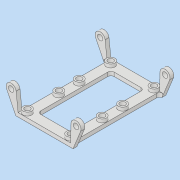
# Autodesk Inventor part: RelayHolderREV2
Saved by Autodesk Inventor 2017.3 (Build 213256000, 256)
## iProperties
Created: 2019-02-24
Part Number: RelayHolderREV2
Material: ABS Plastic
Document SubType Name: Modeling
Designer: Derek Wider
Density: 1.06 g/cm^3
Appearance: Smooth - White
Author: Derek Wider
Autodesk Inventor part; units mm, degrees
ref_plane "YZ Plane" through (0, 0, 0) normal (1, 0, 0) x (0, 1, 0)
ref_plane "XZ Plane" through (0, 0, 0) normal (0, 1, 0) x (-1, 0, 0)
ref_plane "XY Plane" through (0, 0, 0) normal (0, 0, 1) x (1, 0, 0)
sketch "Sketch1" plane through (0, 0, 0) normal (0, 1, 0) x (-1, 0, 0)
  line L0 (0, 0) -> (34, 0)
  line L1 (34, 0) -> (34, -60)
  line L2 (34, -60) -> (0, -60)
  line L3 (0, -60) -> (0, 0)
  dimension "d0" = 34
  dimension "d1" = 60
  constraints: 8 end point, 2 parallel, 1 horizontal, 1 perpendicular
  measures "d0" distance of L1.end L2.end
  measures "d1" distance of L0.end L1.end
extrude "Extrusion1" add sketch "Sketch1" along normal blind 2.5
sketch "Sketch4" plane through (-34, 0, 0) normal (0, 0, 1) x (1, 0, 0)
  circle A0 centre (-4.5, 13.5) radius 1.75
  circle A1 centre (-4.5, 13.5) radius 3.25
  circle A2 centre (37.41, 13.5) radius 1.75
  circle A3 centre (37.41, 13.5) radius 3.25
  line L0 (0, 0) -> (0, 2.5) projected
  line L1 (0, 2.5) -> (34, 2.5) projected
  line L2 (0, 2.5) -> (-1.2701, 13.8611)
  line L3 (34, 0) -> (0, 0) projected
  line L4 (0, 0) -> (-1.5, 0)
  line L5 (-1.5, 0) -> (-7.4181, 12.0691)
  line L6 (34, 2.5) -> (34.1603, 13.5472)
  line L7 (34, 0) -> (35.5, 0)
  line L8 (35.5, 0) -> (40.4267, 12.2908)
  line L9 (34, 0) -> (34, 2.5) projected
  line L10 (34, 2.5) -> (34, 0)
  dimension "d4" = 3.5
  dimension "d5" = 6.5
  dimension "d6" = 4.5
  dimension "d7" = 41.91
  dimension "d8" = 11
  dimension "d9" = 1.5
  dimension "d10" = 1.5
  constraints: 14 end point, 4 centre point, 4 point on circle, 4 tangent, 2 coincident, 2 equal radius, 1 collinear, 1 horizontal, 1 horizontal alignment, 1 point on line
  measures "d4" diameter of A0
  measures "d5" diameter of A1
  measures "d6" distance from line of L0 A0.centre
  measures "d7" distance of A0.centre A2.centre
  measures "d8" distance from line of A0.centre L1
  measures "d9" distance of L0.start L4.end
  measures "d10" distance of L3.start L7.end
extrude "Extrusion2" add sketch "Sketch4" against normal blind 2.5 contours A1 | A1 L2 L0 L4 L5 | L6 A3 L8 L7 L9 | A3
pattern_linear "Rectangular Pattern1" count 2 spacing 57.5 along (0, 0, -1) of "Extrusion2"
hole "Hole1" at (-31, 2.5, -3) direction (0, -1, 0) diameter 3.5 end through all
sketch "Sketch7" plane through (0, 2.5, 0) normal (0, 1, 0) x (1, 0, 0)
  circle A0 centre (-31, 3) radius 1.75 projected
  circle A1 centre (-31, 3) radius 2.75
  point P0 (0, 0)
  dimension "d37" = 5.5
  constraints: 1 centre point, 1 coincident
  measures "d37" diameter of A1
extrude "Extrusion3" add sketch "Sketch7" along normal blind 2.2
pattern_linear "Rectangular Pattern2" count 2 spacing 28 along (1, 0, 0) count 2 spacing 20.3 along (0, 0, -1) of "Hole1", "Extrusion3"
pattern_linear "Rectangular Pattern3" count 2 spacing 33.5 along (0, 0, -1) of "Rectangular Pattern2", "Extrusion3", "Hole1"
sketch "Sketch8" plane through (0, 2.5, 0) normal (0, 1, 0) x (1, 0, 0)
  circle A0 centre (-3, 56.8) radius 2.75 projected
  circle A1 centre (-31, 56.8) radius 2.75 projected
  circle A2 centre (-3, 36.5) radius 2.75 projected
  circle A3 centre (-31, 36.5) radius 2.75 projected
  circle A4 centre (-3, 23.3) radius 2.75 projected
  circle A5 centre (-31, 23.3) radius 2.75 projected
  circle A6 centre (-3, 3) radius 2.75 projected
  circle A7 centre (-31, 3) radius 2.75 projected
  line L0 (-34, 0) -> (0, 0) projected
  line L1 (0, 0) -> (0, 2.5) projected
  line L2 (0, 2.5) -> (0, 57.5) projected
  line L3 (0, 57.5) -> (0, 60) projected
  line L4 (0, 60) -> (-34, 60) projected
  line L5 (-34, 60) -> (-34, 57.5) projected
  line L6 (-34, 57.5) -> (-34, 2.5) projected
  line L7 (-34, 2.5) -> (-34, 0) projected
  line L8 (-27.7, 6.3) -> (-27.7, 53.7)
  line L9 (-27.7, 53.7) -> (-6.3, 53.7)
  line L10 (-6.3, 53.7) -> (-6.3, 6.3)
  line L11 (-6.3, 6.3) -> (-27.7, 6.3)
  dimension "d40" = 6.3
  constraints: 8 end point, 3 other
  measures "d40" distance between parallel lines of L6 L8
extrude "Extrusion4" cut sketch "Sketch8" against normal through all contours L8 L9 L10 L11
fillet "Fillet1" radius 2 8 edges at (-34, 1.25, -2.5) (-34, 1.25, -57.5) (0, 1.25, -57.5) (0, 1.25, -2.5) (-6.3, 1.25, -6.3) (-27.7, 1.25, -6.3) (-27.7, 1.25, -53.7) (-6.3, 1.25, -53.7)
body "Solid1"
